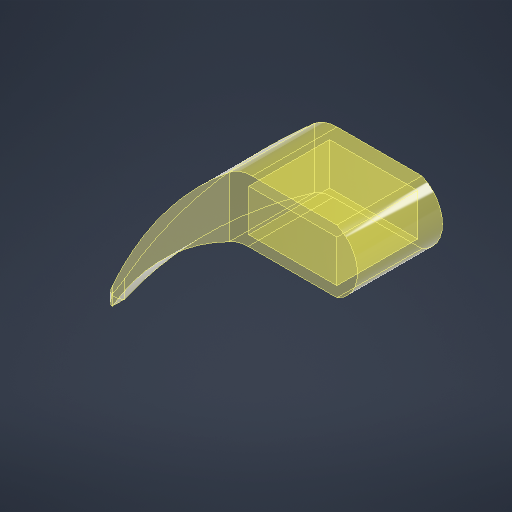
# Autodesk Inventor part: Spider_Robot_Tibia_V1
Saved by Autodesk Inventor 2026.2 (Build 302298010, 298A)
## iProperties
Created: 2026-08-14
Part Number: Spider_Robot_Tibia_V1
Material: Generic
Document SubType Name: Modeling
Designer: Entity
Mass: 75.477 g
Surface Area: 218.516 cm^2
Volume: 75.477 cm^3
Density: 1 g/cm^3
Appearance: Clear - Yellow
Author: Entity
Autodesk Inventor part; units mm, degrees
ref_plane "YZ Plane" through (0, 0, 0) normal (1, 0, 0) x (0, 1, 0)
ref_plane "XZ Plane" through (0, 0, 0) normal (0, 1, 0) x (-1, 0, 0)
ref_plane "XY Plane" through (0, 0, 0) normal (0, 0, 1) x (1, 0, 0)
sketch "Sketch1" plane through (0, 0, 0) normal (0, 0, 1) x (1, 0, 0)
  line L0 (-21, 10) -> (21, 10)
  line L1 (21, 10) -> (21, -10)
  line L2 (21, -10) -> (-21, -10)
  line L3 (-21, -10) -> (-21, 10)
  line L4 (21, 15) -> (-19.3814, 15)
  line L5 (21, -15) -> (-21.3289, -15)
  arc A0 (-30.3889, 10.9551) -> (-106.2021, -86.7378) centre (164.8345, -218.8085) ccw
  arc A1 (-106.2021, -86.7378) -> (-103.2462, -89.2462) centre (-104.4035, -87.6142) ccw
  arc A2 (-30.3302, -17.5786) -> (-103.2462, -89.2462) centre (94.391, -217.3993) ccw
  arc A3 (-19.3814, 15) -> (-30.3889, 10.9551) centre (-19.3814, -2) ccw
  arc A4 (-21.3289, -15) -> (-30.3302, -17.5786) centre (-21.3289, -32) ccw
  arc A5 (21, -15) -> (21, 15) centre (14.4642, 0) ccw
  point P0 (0, 0)
  point P1 (-21, 0)
  point P2 (-26.1005, -15)
  point P3 (-25.5259, 15)
  dimension "d0" = 42
  dimension "d1" = 20
  dimension "d2" = 10
  dimension "d3" = 21
  dimension "d15" = 301.502
  dimension "d16" = 235.5497
  dimension "d17" = 17
  constraints: 14 point on circle, 12 end point, 6 centre point, 5 tangent, 3 horizontal, 2 parallel, 2 point on line, 1 equal radius, 1 midpoint, 1 perpendicular
  measures "d0" distance of L0.start L0.end
  measures "d1" distance of L2.end L0.start
  measures "d2" distance from line of L0 point (0, 0)
  measures "d3" distance of point (-21, 0) point (0, 0)
  measures "d15" radius of A0
  measures "d16" radius of A2
  measures "d17" radius of A3
extrude "Extrusion1" add sketch "Sketch1" along normal blind 40.5 contours L0 L1 L2 L3 | A5 L5 A4 A2 A1 A0 A3 L4
sketch "Sketch2" plane through (-19.3814, 15, 0) normal (0, 1, 0) x (1, 0, 0)
  line L0 (0, 0) -> (0, -40.5) projected
  line L1 (0, -20.25) -> (-86.8207, -20.25)
  line L2 (-86.8207, 0) -> (-86.8207, -40.5) projected
  line L3 (-11.0075, 0) -> (0, 0) projected
  line L4 (-11.0075, -40.5) -> (0, -40.5) projected
  line L5 (-83.8648, 0) -> (-83.8648, -40.5) projected
  line L6 (-83.8648, -20.25) -> (-83.8648, -23.206)
  line L7 (-83.8648, -23.206) -> (-11.0075, -40.5)
  line L8 (-87.0229, 0) -> (-87.0229, -40.5) projected
  arc A0 (-87.0229, -20.25) -> (-83.8648, -23.206) centre (-82.8584, -18.9658) ccw
  line L9 (-83.8648, -17.294) -> (-11.0075, 0)
  arc A1 (-83.8648, -17.294) -> (-87.0229, -20.25) centre (-82.8584, -21.5342) ccw
  line L10 (-11.0075, -40.5) -> (-87.0229, -40.5)
  line L11 (-11.0075, 0) -> (-87.0229, 0)
  line L12 (-87.0229, -40.5) -> (-87.0229, 0)
  point P0 (19.3814, 0)
  dimension "d19" = 2.956
  constraints: 14 end point, 4 midpoint, 4 point on circle, 2 centre point, 2 symmetric about line, 1 horizontal, 1 parallel, 1 perpendicular, 1 point on line, 1 tangent, 1 other
  measures "d19" distance of L6.start L6.end
extrude "Extrusion2" cut sketch "Sketch2" against normal through all contours L9 L5 L11 | A1 L2 L11 L5 | L10 L5 L7 | L5 L10 L2 A0 | A1 L8 L11 L2 | L2 L10 L8 A0
sketch "Sketch3" plane through (0, 0, 40.5) normal (0, 0, 1) x (1, 0, 0)
  line L0 (-21.3289, -15) -> (21, -15) projected
  line L1 (21, 15) -> (21, -15)
  line L2 (21, 0) -> (-21, 0)
  line L3 (-21, 0) -> (-21, 10)
  line L4 (-21, 10) -> (21, 10)
  line L5 (21, 10) -> (21, -10)
  line L6 (21, -10) -> (-21, -10)
  line L7 (-21, -10) -> (-21, 10)
  point P0 (0, 0)
  dimension "d22" = 42
  dimension "d23" = 10
  dimension "d24" = 42
  dimension "d25" = 20
  constraints: 14 end point, 2 horizontal, 2 parallel, 2 perpendicular, 1 midpoint, 1 vertical
  measures "d22" distance of L2.start L2.end
  measures "d23" distance of L2.end L3.end
  measures "d24" distance of L5.end L6.end
  measures "d25" distance of L4.end L5.end
extrude "Extrusion3" cut sketch "Sketch3" against normal blind 38.5
body "Solid1"
